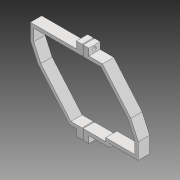
# Autodesk Inventor part: proto_clamp
Saved by Autodesk Inventor 2020 (Build 240168000, 168)
## iProperties
Created: 2021-02-05
Part Number: proto_clamp
Material: Generic
Document SubType Name: Modeling
Designer: DDeGo
Density: 1 g/cm^3
Appearance: Default
Author: DDeGo
Autodesk Inventor part; units mm, degrees
ref_plane "YZ Plane" through (0, 0, 0) normal (1, 0, 0) x (0, 1, 0)
ref_plane "XZ Plane" through (0, 0, 0) normal (0, 1, 0) x (-1, 0, 0)
ref_plane "XY Plane" through (0, 0, 0) normal (0, 0, 1) x (1, 0, 0)
sketch "Sketch1" plane through (0, 0, 0) normal (0, 0, 1) x (1, 0, 0)
  line L0 (56.8649, 0) -> (88.6341, -28.9641)
  line L1 (95.3658, -43.7714) -> (95.3658, -58)
  line L2 (95.3658, -58) -> (69.5112, -58)
  line L3 (69.5112, -58) -> (69.5112, -61)
  line L4 (69.5112, -61) -> (32.5704, -61)
  line L5 (32.5704, -61) -> (6.632, -28.6167)
  line L6 (0, -14.0286) -> (0, 0)
  line L7 (0, 0) -> (56.8649, 0)
  line L8 (55.7026, -3) -> (86.1579, -30.7662)
  line L9 (92.3658, -44.4213) -> (92.3658, -55)
  line L10 (92.3658, -55) -> (66.5112, -55)
  line L11 (66.5112, -55) -> (66.5112, -58)
  line L12 (66.5112, -58) -> (34.0112, -58)
  line L13 (34.0112, -58) -> (9.2079, -27.0338)
  line L14 (3, -13.3787) -> (3, -3)
  line L15 (3, -3) -> (55.7026, -3)
  line L16 (3, -13.3787) -> (8.0044, -24.3866) projected
  line L17 (92.3658, -52.8) -> (92.3658, -44.4213) projected
  line L18 (92.3658, -44.4213) -> (87.3614, -33.4134) projected
  line L19 (66.0112, -57.8) -> (66.0112, -54.8) projected
  line L20 (9.2079, -27.0338) -> (3, -13.3787)
  line L21 (6.632, -28.6167) -> (0, -14.0286)
  line L22 (88.6341, -28.9641) -> (95.3658, -43.7714)
  line L23 (86.1579, -30.7662) -> (92.3658, -44.4213)
  arc A0 (66.4435, -14.9518) -> (47.6829, -3) centre (47.6829, -23.7) ccw projected
  line L24 (34.0112, -57.8) -> (34.0112, -49.6427) projected
  dimension "d0" = 3
  dimension "d2" = 52
  dimension "d3" = 55
  dimension "d27" = 0.5
  dimension "d28" = 15
  dimension "d29" = 3
  dimension "d30" = 3
  dimension "d31" = 3
  dimension "d32" = 15
  dimension "d33" = 3
  dimension "d34" = 3
  constraints: 40 end point, 6 parallel, 6 perpendicular, 3 collinear, 1 horizontal, 1 point on line, 1 tangent, 4 other
  measures "d0" distance between parallel lines of L14 L6
  measures "d2" distance between parallel lines of L10 L15
  measures "d3" distance between parallel lines of L15 L12
  measures "d27" distance between parallel lines of L19 L11
  measures "d28" distance of L13.end L14.start
  measures "d29" distance between parallel lines of L21 L20
  measures "d30" distance between parallel lines of L5 L13
  measures "d31" distance between parallel lines of L4 L12
  measures "d32" distance of L8.end L9.start
  measures "d33" distance between parallel lines of L22 L23
  measures "d34" distance between parallel lines of L0 L8
extrude "Extrusion1" add sketch "Sketch1" along normal blind 10
sketch "Sketch3" plane through (0, 0, 10) normal (0, 0, 1) x (1, 0, 0)
  line L0 (45.6423, 2.3043) -> (46.6423, 2.3043)
  line L1 (46.6423, 2.3043) -> (46.6423, -66.739)
  line L2 (46.6423, -66.739) -> (45.6423, -66.739)
  line L3 (45.6423, -66.739) -> (45.6423, 2.3043)
  point P0 (0, 0)
  dimension "d14" = 1
  constraints: 8 end point, 2 parallel, 1 horizontal, 1 perpendicular
  measures "d14" distance of L0.start L0.end
extrude "Extrusion3" cut sketch "Sketch3" against normal through all
sketch "Sketch4" plane through (0, 0, 10) normal (0, 0, 1) x (1, 0, 0)
  line L0 (45.6423, 0) -> (0, 0) projected
  line L1 (45.6423, 0) -> (40.6423, 0)
  line L2 (40.6423, 0) -> (40.6423, 6)
  line L3 (40.6423, 6) -> (45.6423, 6)
  line L4 (45.6423, 6) -> (45.6423, 0)
  line L5 (56.8649, 0) -> (46.6423, 0) projected
  line L6 (46.6423, 0) -> (51.6423, 0)
  line L7 (51.6423, 0) -> (51.6423, 6)
  line L8 (51.6423, 6) -> (46.6423, 6)
  line L9 (46.6423, 6) -> (46.6423, 0)
  line L10 (45.6423, -61) -> (45.6423, 0) projected
  line L11 (45.6423, -61) -> (40.6423, -61)
  line L12 (40.6423, -61) -> (40.6423, -67)
  line L13 (40.6423, -67) -> (45.6423, -67)
  line L14 (45.6423, -67) -> (45.6423, -61)
  line L15 (46.6423, -61) -> (51.6423, -61)
  line L16 (51.6423, -61) -> (51.6423, -67)
  line L17 (51.6423, -67) -> (46.6423, -67)
  line L18 (46.6423, -67) -> (46.6423, -61)
  point P0 (45.6423, -58)
  dimension "d17" = 6
  dimension "d18" = 5
  constraints: 32 end point, 8 parallel, 5 equal length, 4 horizontal, 4 perpendicular, 4 point on line
  measures "d17" distance of L6.end L7.end
  measures "d18" distance of L2.end L3.end
extrude "Extrusion4" add sketch "Sketch4" against normal up to surface (10 mm away)
sketch "Sketch5" plane through (40.6423, -67, 10) normal (-1, 0, 0) x (0, 0, 1)
  line L0 (0, 0) -> (-10, 0) projected
  line L1 (-5, 0) -> (-5, 73) construction
  line L2 (0, 73) -> (-10, 73) projected
  circle A0 centre (-5, 70) radius 1.6
  circle A1 centre (-5, 3) radius 1.6
  point P0 (-10, 67)
  dimension "d21" = 3
  dimension "d22" = 3
  dimension "d23" = 3.2
  constraints: 2 centre point, 2 end point, 2 midpoint, 2 point on line, 1 equal radius
  measures "d21" distance from line of L2 A0.centre
  measures "d22" distance from line of L0 A1.centre
  measures "d23" diameter of A0
extrude "Extrusion5" cut sketch "Sketch5" against normal through all
equation "\"d29\" = d0"
equation "\"d30\" = d0"
equation "\"d31\" = d0"
equation "\"d33\" = d0"
equation "\"d34\" = d0"
body "Solid1"
